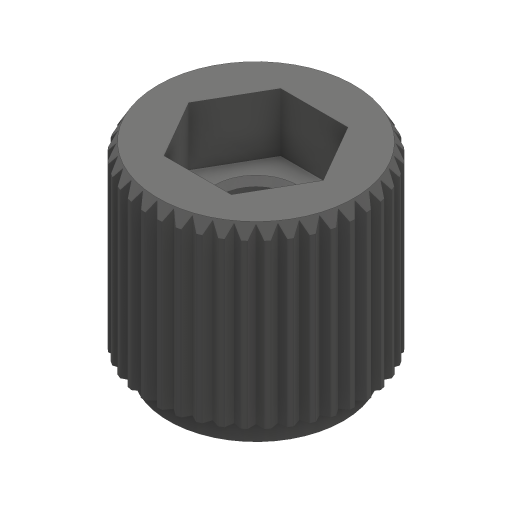
# Autodesk Inventor part: 3DP_ABS_Nut_Knob
Saved by Autodesk Inventor 2024.3 (Build 283343000, 343)
## iProperties
Created: 2018-02-17
Part Number: 3DP_ABS_Nut_Knob
Material: Ogólny
Document SubType Name: Modeling
Designer: Andrzej
Density: 1 g/cm^3
Appearance: Szara
Mass: 3.21202 g
Surface Area: 19.5404 cm^2
Volume: 3.21202 cm^3
Author: Andrzej
Autodesk Inventor part; units mm, degrees
ref_plane "YZ Plane" through (0, 0, 0) normal (1, 0, 0) x (0, 1, 0)
ref_plane "XZ Plane" through (0, 0, 0) normal (0, 1, 0) x (-1, 0, 0)
ref_plane "XY Plane" through (0, 0, 0) normal (0, 0, 1) x (1, 0, 0)
sketch "Szkic1" plane through (0, 0, 0) normal (0, 0, 1) x (1, 0, 0)
  circle A0 centre (0, 0) radius 3.05
  circle A1 centre (0, 0) radius 5
  line L0 (2.8868, 5) -> (5.7735, 0)
  line L1 (5.7735, 0) -> (2.8868, -5)
  line L2 (2.8868, -5) -> (-2.8868, -5)
  line L3 (-2.8868, -5) -> (-5.7735, 0)
  line L4 (-5.7735, 0) -> (-2.8868, 5)
  line L5 (-2.8868, 5) -> (2.8868, 5)
  circle A2 centre (0, 0) radius 7.5
  point P0 (0, 5)
  dimension "d1" = 10
  dimension "d0" = 6.1
  dimension "d2" = 15
  constraints: 12 end point, 4 coincident, 2 centre point, 1 midpoint, 1 vertical alignment, 15 other
  measures "d0" diameter of A0
  measures "d2" diameter of A2
extrude "Wyciągnięcie proste1" add sketch "Szkic1" along normal blind 2 contours A1 | A1 L0 L1 | A1 L5 L0 | L1 L2 A1 | A1 L4 L5 | L2 L3 A1 | A1 L3 L4 | A2
sketch "Szkic2" plane through (0, 0, 2) normal (0, 0, 1) x (1, 0, 0)
  point P0 (0, 0)
sketch "Szkic3" plane through (0, 0, 2) normal (0, 0, 1) x (1, 0, 0)
  circle A0 centre (0, 0) radius 9
  circle A1 centre (0, 0) radius 3.05 projected
  circle A2 centre (0, 0) radius 7.5 projected
  dimension "d7" = 18
  constraints: 1 centre point, 1 coincident
  measures "d7" diameter of A0
extrude "Wyciągnięcie proste4" add sketch "Szkic3" along normal blind 15 contours A0 | A2
sketch "Szkic4" plane through (0, 0, 17) normal (0, 0, 1) x (1, 0, 0)
  circle A0 centre (0, 0) radius 9 projected
  circle A1 centre (0, 0) radius 9 projected
  line L0 (-0.5, 8.9861) -> (0, 8.4861)
  line L1 (-0.5, 8.9861) -> (1.9615, 8.9861) construction
  line L2 (0.5, 8.9861) -> (0, 8.4861)
  line L3 (0.5, 8.9861) -> (4.7976, 8.9861) construction
  dimension "d16" = 45
  dimension "d18" = 135
  dimension "d19" = 0.5
  dimension "d20" = 0.5
  constraints: 8 end point, 2 horizontal, 2 point on circle, 1 point on line, 2 other
  measures "d16" angle of L0 L1
  measures "d18" angle of L2 L3
  measures "d19" horizontal distance of point (0, 0) L0.start
  measures "d20" horizontal distance of point (0, 0) L2.start
extrude "Wyciągnięcie proste5" cut sketch "Szkic4" against normal blind 15 contours L2 L0 A0 picked at (0.2222, 8.8236)
pattern_circular "Szyk kołowy1" count 40 over 360 about axis through (0, 0, -10) along (0, 0, 1) of "Wyciągnięcie proste5"
fillet "Zaokrąglenie1" radius 0.8 1 edges at (-7.5, 0, 2)
sketch "Szkic6" plane through (0, 0, 17) normal (0, 0, 1) x (1, 0, 0)
  line L0 (1.3275, 8.3816) -> (0.9119, 8.9537) projected
  arc A0 (0.9119, 8.9537) -> (0.5, 8.9861) centre (0, 0) ccw projected
  line L1 (0.5, 8.9861) -> (0, 8.4861) projected
  line L2 (0, 8.4861) -> (-0.5, 8.9861) projected
  arc A1 (-0.5, 8.9861) -> (-0.9119, 8.9537) centre (0, 0) ccw projected
  line L3 (-0.9119, 8.9537) -> (-1.3275, 8.3816) projected
  line L4 (-1.3275, 8.3816) -> (-1.8996, 8.7972) projected
  arc A2 (-1.8996, 8.7972) -> (-2.3013, 8.7008) centre (0, 0) ccw projected
  line L5 (-2.3013, 8.7008) -> (-2.6223, 8.0708) projected
  line L6 (-2.6223, 8.0708) -> (-3.2524, 8.3918) projected
  arc A3 (-3.2524, 8.3918) -> (-3.6341, 8.2337) centre (0, 0) ccw projected
  line L7 (-3.6341, 8.2337) -> (-3.8526, 7.5612) projected
  line L8 (-3.8526, 7.5612) -> (-4.5251, 7.7797) projected
  arc A4 (-4.5251, 7.7797) -> (-4.8774, 7.5638) centre (0, 0) ccw projected
  line L9 (-4.8774, 7.5638) -> (-4.988, 6.8654) projected
  line L10 (-4.988, 6.8654) -> (-5.6864, 6.976) projected
  arc A5 (-5.6864, 6.976) -> (-6.0006, 6.7077) centre (0, 0) ccw projected
  line L11 (-6.0006, 6.7077) -> (-6.0006, 6.0006) projected
  line L12 (-6.0006, 6.0006) -> (-6.7077, 6.0006) projected
  arc A6 (-6.7077, 6.0006) -> (-6.976, 5.6864) centre (0, 0) ccw projected
  line L13 (-6.976, 5.6864) -> (-6.8654, 4.988) projected
  line L14 (-6.8654, 4.988) -> (-7.5638, 4.8774) projected
  arc A7 (-7.5638, 4.8774) -> (-7.7797, 4.5251) centre (0, 0) ccw projected
  line L15 (-7.7797, 4.5251) -> (-7.5612, 3.8526) projected
  line L16 (-7.5612, 3.8526) -> (-8.2337, 3.6341) projected
  arc A8 (-8.2337, 3.6341) -> (-8.3918, 3.2524) centre (0, 0) ccw projected
  line L17 (-8.3918, 3.2524) -> (-8.0708, 2.6223) projected
  line L18 (-8.0708, 2.6223) -> (-8.7008, 2.3013) projected
  arc A9 (-8.7008, 2.3013) -> (-8.7972, 1.8996) centre (0, 0) ccw projected
  line L19 (-8.7972, 1.8996) -> (-8.3816, 1.3275) projected
  line L20 (-8.3816, 1.3275) -> (-8.9537, 0.9119) projected
  arc A10 (-8.9537, 0.9119) -> (-8.9861, 0.5) centre (0, 0) ccw projected
  line L21 (-8.9861, 0.5) -> (-8.4861, 0) projected
  line L22 (-8.4861, 0) -> (-8.9861, -0.5) projected
  arc A11 (-8.9861, -0.5) -> (-8.9537, -0.9119) centre (0, 0) ccw projected
  line L23 (-8.9537, -0.9119) -> (-8.3816, -1.3275) projected
  line L24 (-8.3816, -1.3275) -> (-8.7972, -1.8996) projected
  arc A12 (-8.7972, -1.8996) -> (-8.7008, -2.3013) centre (0, 0) ccw projected
  line L25 (-8.7008, -2.3013) -> (-8.0708, -2.6223) projected
  line L26 (-8.0708, -2.6223) -> (-8.3918, -3.2524) projected
  arc A13 (-8.3918, -3.2524) -> (-8.2337, -3.6341) centre (0, 0) ccw projected
  line L27 (-8.2337, -3.6341) -> (-7.5612, -3.8526) projected
  line L28 (-7.5612, -3.8526) -> (-7.7797, -4.5251) projected
  arc A14 (-7.7797, -4.5251) -> (-7.5638, -4.8774) centre (0, 0) ccw projected
  line L29 (-7.5638, -4.8774) -> (-6.8654, -4.988) projected
  line L30 (-6.8654, -4.988) -> (-6.976, -5.6864) projected
  arc A15 (-6.976, -5.6864) -> (-6.7077, -6.0006) centre (0, 0) ccw projected
  line L31 (-6.7077, -6.0006) -> (-6.0006, -6.0006) projected
  line L32 (-6.0006, -6.0006) -> (-6.0006, -6.7077) projected
  arc A16 (-6.0006, -6.7077) -> (-5.6864, -6.976) centre (0, 0) ccw projected
  line L33 (-5.6864, -6.976) -> (-4.988, -6.8654) projected
  line L34 (-4.988, -6.8654) -> (-4.8774, -7.5638) projected
  arc A17 (-4.8774, -7.5638) -> (-4.5251, -7.7797) centre (0, 0) ccw projected
  line L35 (-4.5251, -7.7797) -> (-3.8526, -7.5612) projected
  line L36 (-3.8526, -7.5612) -> (-3.6341, -8.2337) projected
  arc A18 (-3.6341, -8.2337) -> (-3.2524, -8.3918) centre (0, 0) ccw projected
  line L37 (-3.2524, -8.3918) -> (-2.6223, -8.0708) projected
  line L38 (-2.6223, -8.0708) -> (-2.3013, -8.7008) projected
  arc A19 (-2.3013, -8.7008) -> (-1.8996, -8.7972) centre (0, 0) ccw projected
  line L39 (-1.8996, -8.7972) -> (-1.3275, -8.3816) projected
  line L40 (-1.3275, -8.3816) -> (-0.9119, -8.9537) projected
  arc A20 (-0.9119, -8.9537) -> (-0.5, -8.9861) centre (0, 0) ccw projected
  line L41 (-0.5, -8.9861) -> (0, -8.4861) projected
  line L42 (0, -8.4861) -> (0.5, -8.9861) projected
  arc A21 (0.5, -8.9861) -> (0.9119, -8.9537) centre (0, 0) ccw projected
  line L43 (0.9119, -8.9537) -> (1.3275, -8.3816) projected
  line L44 (1.3275, -8.3816) -> (1.8996, -8.7972) projected
  arc A22 (1.8996, -8.7972) -> (2.3013, -8.7008) centre (0, 0) ccw projected
  line L45 (2.3013, -8.7008) -> (2.6223, -8.0708) projected
  line L46 (2.6223, -8.0708) -> (3.2524, -8.3918) projected
  arc A23 (3.2524, -8.3918) -> (3.6341, -8.2337) centre (0, 0) ccw projected
  line L47 (3.6341, -8.2337) -> (3.8526, -7.5612) projected
  line L48 (3.8526, -7.5612) -> (4.5251, -7.7797) projected
  arc A24 (4.5251, -7.7797) -> (4.8774, -7.5638) centre (0, 0) ccw projected
  line L49 (4.8774, -7.5638) -> (4.988, -6.8654) projected
  line L50 (4.988, -6.8654) -> (5.6864, -6.976) projected
  arc A25 (5.6864, -6.976) -> (6.0006, -6.7077) centre (0, 0) ccw projected
  line L51 (6.0006, -6.7077) -> (6.0006, -6.0006) projected
  line L52 (6.0006, -6.0006) -> (6.7077, -6.0006) projected
  arc A26 (6.7077, -6.0006) -> (6.976, -5.6864) centre (0, 0) ccw projected
  line L53 (6.976, -5.6864) -> (6.8654, -4.988) projected
  line L54 (6.8654, -4.988) -> (7.5638, -4.8774) projected
  arc A27 (7.5638, -4.8774) -> (7.7797, -4.5251) centre (0, 0) ccw projected
  line L55 (7.7797, -4.5251) -> (7.5612, -3.8526) projected
  line L56 (7.5612, -3.8526) -> (8.2337, -3.6341) projected
  arc A28 (8.2337, -3.6341) -> (8.3918, -3.2524) centre (0, 0) ccw projected
  line L57 (8.3918, -3.2524) -> (8.0708, -2.6223) projected
  line L58 (8.0708, -2.6223) -> (8.7008, -2.3013) projected
  arc A29 (8.7008, -2.3013) -> (8.7972, -1.8996) centre (0, 0) ccw projected
  line L59 (8.7972, -1.8996) -> (8.3816, -1.3275) projected
  line L60 (8.3816, -1.3275) -> (8.9537, -0.9119) projected
  arc A30 (8.9537, -0.9119) -> (8.9861, -0.5) centre (0, 0) ccw projected
  line L61 (8.9861, -0.5) -> (8.4861, 0) projected
  line L62 (8.4861, 0) -> (8.9861, 0.5) projected
  arc A31 (8.9861, 0.5) -> (8.9537, 0.9119) centre (0, 0) ccw projected
  line L63 (8.9537, 0.9119) -> (8.3816, 1.3275) projected
  line L64 (8.3816, 1.3275) -> (8.7972, 1.8996) projected
  arc A32 (8.7972, 1.8996) -> (8.7008, 2.3013) centre (0, 0) ccw projected
  line L65 (8.7008, 2.3013) -> (8.0708, 2.6223) projected
  line L66 (8.0708, 2.6223) -> (8.3918, 3.2524) projected
  arc A33 (8.3918, 3.2524) -> (8.2337, 3.6341) centre (0, 0) ccw projected
  line L67 (8.2337, 3.6341) -> (7.5612, 3.8526) projected
  line L68 (7.5612, 3.8526) -> (7.7797, 4.5251) projected
  arc A34 (7.7797, 4.5251) -> (7.5638, 4.8774) centre (0, 0) ccw projected
  line L69 (7.5638, 4.8774) -> (6.8654, 4.988) projected
  line L70 (6.8654, 4.988) -> (6.976, 5.6864) projected
  arc A35 (6.976, 5.6864) -> (6.7077, 6.0006) centre (0, 0) ccw projected
  line L71 (6.7077, 6.0006) -> (6.0006, 6.0006) projected
  line L72 (6.0006, 6.0006) -> (6.0006, 6.7077) projected
  arc A36 (6.0006, 6.7077) -> (5.6864, 6.976) centre (0, 0) ccw projected
  line L73 (5.6864, 6.976) -> (4.988, 6.8654) projected
  line L74 (4.988, 6.8654) -> (4.8774, 7.5638) projected
  arc A37 (4.8774, 7.5638) -> (4.5251, 7.7797) centre (0, 0) ccw projected
  line L75 (4.5251, 7.7797) -> (3.8526, 7.5612) projected
  line L76 (3.8526, 7.5612) -> (3.6341, 8.2337) projected
  arc A38 (3.6341, 8.2337) -> (3.2524, 8.3918) centre (0, 0) ccw projected
  line L77 (3.2524, 8.3918) -> (2.6223, 8.0708) projected
  line L78 (2.6223, 8.0708) -> (2.3013, 8.7008) projected
  arc A39 (2.3013, 8.7008) -> (1.8996, 8.7972) centre (0, 0) ccw projected
  line L79 (1.8996, 8.7972) -> (1.3275, 8.3816) projected
  circle A40 centre (0, 0) radius 3.05 projected
  circle A41 centre (0, 0) radius 5
  line L80 (-2.8868, -5) -> (-5.7735, 0)
  line L81 (-5.7735, 0) -> (-2.8868, 5)
  line L82 (-2.8868, 5) -> (2.8868, 5)
  line L83 (2.8868, 5) -> (5.7735, 0)
  line L84 (5.7735, 0) -> (2.8868, -5)
  line L85 (2.8868, -5) -> (-2.8868, -5)
  point P0 (0, -5)
  dimension "d30" = 10
  constraints: 12 end point, 2 coincident, 1 midpoint, 1 vertical alignment, 15 other
extrude "Wyciągnięcie proste6" cut sketch "Szkic6" against normal blind 5 contours A41 | A41 L83 L84 | A41 L82 L83 | L84 L85 A41 | A41 L81 L82 | L85 L80 A41 | A41 L80 L81
chamfer "Faza2" distance 0.5 angle 45 2 edges at (-3.05, 0, 12) (-3.05, 0, 0)
sketch "Szkic7" plane through (0, 0, 0) normal (0, 1, 0) x (-1, 0, 0)
  line L0 (-9.7062, 14.7416) -> (-7.4452, 18.6578)
  line L1 (-9.7062, 14.7416) -> (-5.1842, 14.7416) construction
  line L2 (-7.4452, 18.6578) -> (-11.5433, 18.6578)
  line L3 (-11.5433, 18.6578) -> (-9.7062, 14.7416)
  line L4 (0, -3.629) -> (0, 21.7738) projected
  point P0 (0, 0)
  dimension "d36" = 4.522
  dimension "d37" = 60
  constraints: 8 end point, 2 horizontal, 1 equal length
  measures "d36" distance of L0.start L0.end
  measures "d37" angle of L1 L0
revolve "Obrót2" cut sketch "Szkic7" angle 360 about axis through (0, 0, -10) along (0, 0, 1)
